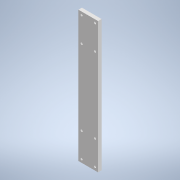
# Autodesk Inventor part: side upper and lower connector
Saved by Autodesk Inventor 2021 (Build 250183000, 183)
## iProperties
Created: 2021-11-20
Part Number: side upper and lower connector
Material: Generic
Document SubType Name: Modeling
Designer: techv
Density: 1 g/cm^3
Appearance: Default
Author: techv
Autodesk Inventor part; units mm, degrees
ref_plane "YZ Plane" through (0, 0, 0) normal (1, 0, 0) x (0, 1, 0)
ref_plane "XZ Plane" through (0, 0, 0) normal (0, 1, 0) x (-1, 0, 0)
ref_plane "XY Plane" through (0, 0, 0) normal (0, 0, 1) x (1, 0, 0)
sketch "Sketch1" plane through (0, 0, 0) normal (0, 0, 1) x (1, 0, 0)
  line L0 (15, 43) -> (43, 43) projected
  line L1 (15, 1) -> (15, 43) projected
  line L2 (43, 1) -> (15, 1) projected
  line L3 (43, 1) -> (43, 43) projected
  line L4 (15, 187) -> (43, 187) projected
  line L5 (15, 145) -> (15, 187) projected
  line L6 (43, 145) -> (15, 145) projected
  line L7 (43, 145) -> (43, 187) projected
  line L8 (15, 187) -> (43, 187)
  line L9 (43, 187) -> (43, 1)
  line L10 (43, 1) -> (15, 1)
  line L11 (15, 1) -> (15, 187)
  point P0 (0, 0)
  constraints: 8 end point, 2 parallel, 1 horizontal, 1 perpendicular
extrude "Extrusion1" add sketch "Sketch1" along normal blind 5
sketch "Sketch2" plane through (0, 0, 5) normal (0, 0, 1) x (1, 0, 0)
  line L0 (43, 1) -> (43, 187) projected
  line L1 (43, 187) -> (15, 187) projected
  line L2 (15, 187) -> (15, 1) projected
  line L3 (15, 1) -> (43, 1) projected
  line L4 (15, 187) -> (15, 1) construction
  line L5 (15, 5.5) -> (43, 5.5) construction
  line L6 (43, 1) -> (43, 187) construction
  line L7 (15, 1) -> (43, 1) construction
  line L8 (19.5, 1) -> (19.5, 187) construction
  line L9 (43, 187) -> (15, 187) construction
  circle A0 centre (19.5, 5.5) radius 1.5
  line L10 (43, 45) -> (15, 45) projected
  circle A1 centre (38.5, 5.5) radius 1.5
  circle A2 centre (19.5, 40.5) radius 1.5
  circle A3 centre (38.5, 40.5) radius 1.5
  circle A4 centre (19.5, 182.5) radius 1.5
  circle A5 centre (19.5, 147.5) radius 1.5
  circle A6 centre (38.5, 147.5) radius 1.5
  circle A7 centre (38.5, 182.5) radius 1.5
  point P0 (0, 0)
  dimension "d2" = 4.5
  dimension "d3" = 4.5
  dimension "d4" = 3
  dimension "d5" = 44
  dimension "d6" = 28
  dimension "d9" = 19
  dimension "d12" = 35
  dimension "d15" = 186
  dimension "d18" = 142
  constraints: 8 centre point, 6 point on line, 4 end point, 2 perpendicular, 2 vertical, 1 horizontal, 14 other
  measures "d2" distance between parallel lines of L2 L8
  measures "d3" distance between parallel lines of L3 L5
  measures "d4" diameter of A0
  measures "d5" distance between parallel lines of L3 L10
  measures "d6" distance of L2.end L0.start
  measures "d9" distance of A0.centre A1.centre
  measures "d12" distance of A0.centre A2.centre
  measures "d15" distance between parallel lines of L1 L3
  measures "d18" distance of A2.centre A4.centre
extrude "Extrusion2" cut sketch "Sketch2" against normal through all contours A0 | A1 | A2 | A3 | A4 | A5 | A6 | A7
body "Solid1"
